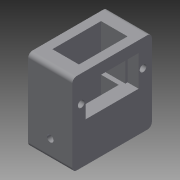
# Autodesk Inventor part: soporte-servo-valvula
Saved by Autodesk Inventor 2015 SP1 (Build 190203100, 203)
## iProperties
Created: 2015-07-03
Part Number: soporte-servo-valvula
Material: Genérico
Document SubType Name: Modeling
Designer: Javier
Density: 1 g/cm^3
Appearance: Valor por defecto
Author: Javier
Autodesk Inventor part; units mm, degrees
ref_plane "YZ Plane" through (0, 0, 0) normal (1, 0, 0) x (0, 1, 0)
ref_plane "XZ Plane" through (0, 0, 0) normal (0, 1, 0) x (-1, 0, 0)
sketch "Boceto1" plane through (0, 0, 0) normal (0, 0, 1) x (1, 0, 0)
  point P0 (0, 0)
sketch "Boceto2" plane through (0, 0, 0) normal (0, 0, 1) x (1, 0, 0)
  circle A0 centre (5, -10) radius 2 projected
  line L0 (0, -20) -> (0, 0) projected
  line L1 (0, -20) -> (10, -20) projected
  line L2 (10, 0) -> (10, -20) projected
  line L3 (0, 0) -> (10, 0) projected
  line L4 (0, -20) -> (10, -20)
  line L5 (10, -20) -> (10, 0)
  line L6 (10, 0) -> (0, 0)
  line L7 (0, 0) -> (0, -20)
  line L8 (0, -20) -> (10, 0) construction
  line L9 (10, -20) -> (0, 0) construction
  line L10 (-5, -28) -> (15, -28)
  line L11 (15, -28) -> (15, 8)
  line L12 (15, 8) -> (-5, 8)
  line L13 (-5, 8) -> (-5, -28)
  line L14 (-5, -28) -> (15, 8) construction
  line L15 (15, -28) -> (-5, 8) construction
  dimension "d0" = 10
  dimension "d1" = 20
  dimension "d2" = 20
  dimension "d3" = 36
  constraints: 24 end point, 4 midpoint, 4 parallel, 2 horizontal, 2 perpendicular
  measures "d0" distance of L6.end L5.end
  measures "d1" distance of L5.end L4.end
  measures "d2" distance of L12.end L11.end
  measures "d3" distance of L11.end L10.end
extrude "Extrusión1" add sketch "Boceto2" against normal blind 15 contours L13 L12 L11 L10
sketch "Boceto3" plane through (0, 0, 0) normal (0, 0, 1) x (1, 0, 0)
  line L0 (10, 0) -> (10, -20) projected
  line L1 (10, -20) -> (0, -20) projected
  line L2 (0, -20) -> (0, 0) projected
  line L3 (0, 0) -> (10, 0) projected
  line L4 (-5, -28) -> (15, -28) projected
  line L5 (15, -28) -> (15, 8) projected
  line L6 (15, 8) -> (-5, 8) projected
  line L7 (-5, 8) -> (-5, -28) projected
  point P0 (0, 0)
  point P1 (5, -10)
extrude "Extrusión2" add sketch "Boceto3" along normal blind 22
sketch "Boceto4" plane through (15, -28, -15) normal (1, 0, 0) x (0, 0, -1)
  line L0 (0, 0) -> (-37, 0) projected
  line L1 (0, 36) -> (0, 0) projected
  line L2 (0, 36) -> (-37, 36) projected
  line L3 (-37, 0) -> (-37, 36) projected
  line L4 (-37, 36) -> (-32, 36)
  line L5 (-32, 36) -> (-32, 0)
  line L6 (-37, 0) -> (0, 0) projected
  line L7 (-32, 18) -> (-32, 30)
  line L8 (-32, 30) -> (-18, 30)
  line L9 (-18, 30) -> (-18, 6)
  line L10 (-18, 6) -> (-32, 6)
  point P0 (-15, 28)
  dimension "d8" = 5
  dimension "d9" = 12
  dimension "d10" = 14
  dimension "d11" = 24
  constraints: 12 end point, 4 point on line, 3 perpendicular, 1 horizontal, 1 midpoint
  measures "d8" distance of L2.end L4.end
  measures "d9" distance of L7.start L7.end
  measures "d10" distance of L7.end L8.end
  measures "d11" distance of L8.end L9.end
extrude "Extrusión3" cut sketch "Boceto4" against normal blind 5 contours L5 L8 L9 L10
sketch "Boceto5" plane through (15, -28, -15) normal (1, 0, 0) x (0, 0, -1)
  line L0 (-32, 30) -> (-18, 30) projected
  line L1 (-18, 6) -> (-32, 6) projected
  line L2 (-25, 30) -> (-25, 32)
  circle A0 centre (-25, 32) radius 1.5
  line L3 (-18, 6) -> (-32, 6) projected
  line L4 (-25, 6) -> (-25, 4)
  circle A1 centre (-25, 4) radius 1.5
  point P0 (-15, 28)
  dimension "d14" = 2
  dimension "d15" = 3
  dimension "d16" = 2
  dimension "d17" = 3
  constraints: 4 end point, 2 centre point, 2 coincident, 2 midpoint, 2 vertical
  measures "d14" distance of L2.start L2.end
  measures "d15" diameter of A0
  measures "d16" distance of L4.start L4.end
  measures "d17" diameter of A1
extrude "Extrusión4" cut sketch "Boceto5" against normal blind 15
fillet "Empalme1" radius 2 4 edges at (5, 8, 22) (5, 8, -15) (5, -28, -15) (5, -28, 22)
sketch "Boceto7" plane through (0, -20, -15) normal (1, 0, 0) x (0, 0, -1)
  point P0 (-15, 20)
sketch "Boceto8" plane through (0, 0, 22) normal (0, 0, 1) x (1, 0, 0)
  line L0 (10, -20) -> (0, -20) projected
  line L1 (0, -20) -> (0, 0) projected
  line L2 (0, 0) -> (10, 0) projected
  line L3 (10, 0) -> (10, -20) projected
  line L4 (15, -26) -> (-5, -26) projected
  line L5 (15, -26) -> (15, 6) projected
  line L6 (-5, 6) -> (15, 6) projected
  line L7 (-5, 6) -> (-5, -26) projected
  line L8 (10, 0) -> (10, -20) projected
  line L9 (0, -20) -> (10, -20) projected
  line L10 (1, -1) -> (9, -1)
  line L11 (9, -1) -> (9, -19)
  line L12 (9, -19) -> (1, -19)
  line L13 (1, -19) -> (1, -1)
  line L14 (1, -1) -> (9, -19) construction
  line L15 (9, -1) -> (1, -19) construction
  point P0 (5, -10)
  dimension "d32" = 8
  dimension "d33" = 18
  constraints: 12 end point, 2 midpoint, 2 parallel, 1 horizontal, 1 perpendicular, 1 point on line
  measures "d32" distance of L11.end L12.end
  measures "d33" distance of L10.end L11.end
ref_plane "Plano de trabajo1" through (0, -20, 0) normal (0, 0, 1) x (1, 0, 0)
extrude "Extrusión6" add sketch "Boceto8" against normal up to surface (22 mm away) contours L0 L1 L2 L3
sketch "Boceto9" plane through (0, 0, 22) normal (0, 0, 1) x (1, 0, 0)
  line L0 (10, -20) -> (10, 0) projected
  line L1 (10, 0) -> (0, 0) projected
  line L2 (0, 0) -> (0, -20) projected
  line L3 (0, -20) -> (10, -20) projected
  line L4 (-5, -26) -> (15, -26) projected
  line L5 (-5, -26) -> (-5, 6) projected
  line L6 (15, 6) -> (-5, 6) projected
  line L7 (15, 6) -> (15, -26) projected
  point P0 (0, 0)
extrude "Extrusión7" cut sketch "Boceto9" against normal up to surface (19 mm away) contours L3 L2 L1 L0
sketch "Boceto10" plane through (15, -26, -15) normal (1, 0, 0) x (0, 0, -1)
  circle A0 centre (-25, 30) radius 1.5 projected
  circle A1 centre (-25, 2) radius 1.5 projected
  line L0 (-18, 4) -> (-32, 4) projected
  line L1 (-32, 4) -> (-32, 28) projected
  line L2 (-32, 28) -> (-18, 28) projected
  line L3 (-18, 28) -> (-18, 4) projected
  arc A2 (-37, 0) -> (-35, -2) centre (-35, 0) ccw projected
  line L4 (-2, -2) -> (-35, -2) projected
  arc A3 (-2, -2) -> (0, 0) centre (-2, 0) ccw projected
  line L5 (0, 32) -> (0, 0) projected
  arc A4 (0, 32) -> (-2, 34) centre (-2, 32) ccw projected
  line L6 (-2, 34) -> (-35, 34) projected
  arc A5 (-35, 34) -> (-37, 32) centre (-35, 32) ccw projected
  line L7 (-37, 0) -> (-37, 32) projected
  line L8 (-35, -2) -> (-2, -2) projected
  line L9 (-32, -2) -> (-32, 34)
  point P0 (-15, 26)
  constraints: 2 end point, 2 point on line, 1 perpendicular
extrude "Extrusión8" cut sketch "Boceto10" against normal blind 20 contours L9 L4 A2 L7 A5 L6 L1
sketch "Boceto11" plane through (0, -20, 3) normal (1, 0, 0) x (0, 0, -1)
  line L0 (-14, 20) -> (-14, 0) projected
  line L1 (-14, 0) -> (0, 0) projected
  line L2 (0, 20) -> (0, 0) projected
  line L3 (-14, 20) -> (0, 20) projected
  point P0 (3, 20)
extrude "Extrusión9" cut sketch "Boceto11" against normal blind 20
sketch "Boceto12" plane through (15, -28, 17) normal (0, 0, 1) x (1, 0, 0)
  line L0 (-5, 8) -> (-5, 28) projected
  line L1 (-5, 28) -> (-15, 28) projected
  line L2 (-15, 28) -> (-15, 8) projected
  line L3 (-15, 8) -> (-5, 8) projected
  line L4 (-20, 2) -> (0, 2) projected
  line L5 (-20, 2) -> (-20, 34) projected
  line L6 (0, 34) -> (-20, 34) projected
  line L7 (0, 34) -> (0, 2) projected
  line L8 (0, 0) -> (-20, 0) projected
  line L9 (-15, 0) -> (-15, 36)
  line L10 (-20, 36) -> (0, 36) projected
  line L11 (-15, 36) -> (-20, 36)
  line L12 (-20, 36) -> (-20, 0)
  line L13 (-20, 0) -> (-15, 0)
  point P0 (-15, 28)
  constraints: 8 end point, 2 collinear, 2 point on line, 1 perpendicular, 1 vertical
extrude "Extrusión10" cut sketch "Boceto12" against normal blind 50 contours L9 L4 L5 L6 L2 | L9 L8 L12 L4 | L6 L12 L10 L9
